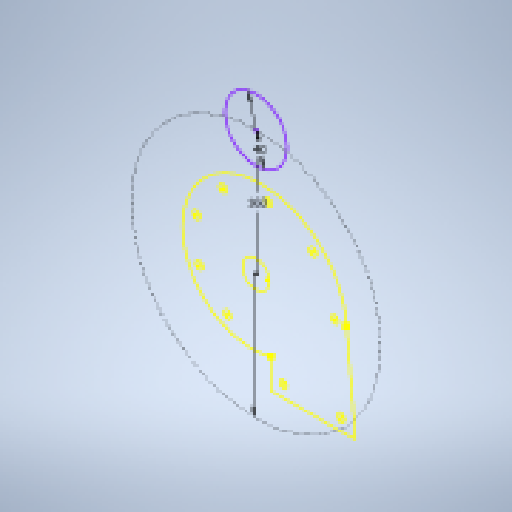
# Autodesk Inventor part: Soporte motor
Saved by Autodesk Inventor 2025.3 (Build 293356000, 356)
## iProperties
Created: 2025-11-12
Part Number: Soporte motor
Material: Generic
Document SubType Name: Modeling
Designer: juanm
Density: 1 g/cm^3
Appearance: Default
Author: juanm
Autodesk Inventor part; units mm, degrees
ref_plane "YZ Plane" through (0, 0, 0) normal (1, 0, 0) x (0, 1, 0)
ref_plane "XZ Plane" through (0, 0, 0) normal (0, 1, 0) x (-1, 0, 0)
ref_plane "XY Plane" through (0, 0, 0) normal (0, 0, 1) x (1, 0, 0)
sketch "Sketch1" plane through (0, 0, 0) normal (0, 0, 1) x (1, 0, 0)
  circle A0 centre (-25.0838, -31.7051) radius 2.5 projected
  circle A1 centre (-43.012, -13.2629) radius 2.5 projected
  circle A2 centre (-44.8914, 13.7567) radius 2.5 projected
  circle A3 centre (-28.0838, 36.7109) radius 2.5 projected
  circle A4 centre (0.8935, 43.7288) radius 2.5 projected
  circle A5 centre (29.5533, 30.4373) radius 2.5 projected
  circle A6 centre (43.6662, -0.0951) radius 2.5 projected
  circle A7 centre (47.6662, -52.5951) radius 2.5 projected
  circle A8 centre (10.6662, -52.5951) radius 2.5 projected
  circle A9 centre (-6.8338, -0.0951) radius 8.75 projected
  line L0 (56.6662, -60.0951) -> (51.1662, -0.0951) projected
  spline S0 degree 4 poles (51.1662, -0.0951) (50.0319, 24.6801) (26.25, 55.8136) (-25.1104, 60.0951) (-56.6662, 18.5311) (-54.7055, -22.2338) (-29.645, -43.1708) (-8.3823, -44.3792) (3.1662, -40.8213) knots 0 0 0 0 0 0.330099 0.457579 0.582312 0.704438 0.895347 0.895347 0.895347 0.895347 0.895347 projected
  line L1 (3.1662, -40.8213) -> (3.1662, -60.0951) projected
  line L2 (3.1662, -60.0951) -> (56.6662, -60.0951) projected
  circle A10 centre (-6.8338, -0.0951) radius 80 construction
  circle A11 centre (-6.745, 79.9048) radius 20
  spline S1 degree 4 poles (13.255, 79.9049) (13.2551, 61.5553) (53.2021, 31.1275) (45.8959, 8.6921) (-3.4008, 37.4416) (-15.4753, 22.3192) (-58.9134, 17.0029) (-26.745, 63.4724) (-26.745, 79.9049) knots 0 0 0 0 0 0.269013 0.429481 0.564366 0.732064 1 1 1 1 1
  point P0 (0, 0)
  point P1 (42.4397, 26.511)
  point P2 (35.1236, 20.7708)
  point P3 (0.8932, 30.4369)
  point P4 (-17.5374, 26.5111)
  point P5 (-37.1432, 26.5121)
  dimension "d0" = 160
  dimension "d1" = 40
  constraints: 2 point on circle, 1 centre point, 1 coincident, 12 other
  measures "d1" diameter of A11
extrude "Extrusion1" add sketch "Sketch1" along normal blind 5 contours S1 S0 | S0 S1 A11 | A11
body "Solid1"
